Autodesk Inventor part; units mm, degrees
(part 3 of 3)
  line L372 (-9.4727, -16.9965) -> (-8.9155, -16.4393) projected
  line L373 (-10.552, -17.5763) -> (-10.5765, -17.5519) projected
  line L374 (-10.5765, -17.5519) -> (-10.9223, -17.8977) projected
  line L375 (-13.8024, -11.0005) -> (-15.4197, -12.6178) projected
  line L376 (-15.4197, -12.6178) -> (-15.1472, -12.8903) projected
  line L377 (-15.1472, -12.8903) -> (-13.5299, -11.273) projected
  line L378 (-13.5299, -11.273) -> (-13.8024, -11.0005) projected
  line L379 (-16.2092, -10.5708) -> (-15.3551, -11.4249) projected
  line L380 (-15.5559, -9.4461) -> (-15.8529, -9.743) projected
  line L381 (-15.8529, -9.743) -> (-15.8371, -9.7587) projected
  line L382 (-15.1472, -11.2171) -> (-16.2668, -10.0975) projected
  line L383 (-16.2668, -10.0975) -> (-16.4152, -10.246) projected
  line L384 (-16.0397, -8.7632) -> (-18.2911, -11.0145) projected
  line L385 (-18.2911, -11.0145) -> (-18.0186, -11.2869) projected
  line L386 (-18.0186, -11.2869) -> (-15.7673, -9.0356) projected
  line L387 (-15.7673, -9.0356) -> (-16.0397, -8.7632) projected
  circle A0 centre (-12.4372, -30.0261) radius 2.75 projected
  circle A1 centre (12.4372, -30.0261) radius 2.75 projected
  circle A2 centre (30.0261, -12.4372) radius 2.75 projected
  circle A3 centre (30.0261, 12.4372) radius 2.75 projected
  circle A4 centre (12.4372, 30.0261) radius 2.75 projected
  circle A5 centre (-22.981, 22.981) radius 2.75 projected
  circle A6 centre (-32.5, 0) radius 2.75 projected
  circle A7 centre (0, 32.5) radius 2.75 projected
  circle A8 centre (-30.0261, -12.4372) radius 2.75 projected
  circle A9 centre (-30.0261, 12.4372) radius 2.75 projected
  circle A10 centre (-12.4372, 30.0261) radius 2.75 projected
  circle A11 centre (22.981, 22.981) radius 2.75 projected
  circle A12 centre (32.5, 0) radius 2.75 projected
  circle A13 centre (22.981, -22.981) radius 2.75 projected
  circle A14 centre (0, -32.5) radius 2.75 projected
  circle A15 centre (-22.981, -22.981) radius 2.75 projected
  circle A16 centre (8, 0) radius 2.1 projected
  circle A17 centre (-8, 0) radius 2.1 projected
  circle A18 centre (0, -8) radius 2.1 projected
  circle A19 centre (0, 8) radius 2.1 projected
  circle A20 centre (0, 0) radius 40 projected
  point P0 (-18.4989, -9.1823)
  point P1 (-18.6788, -8.7509)
  point P2 (-18.0483, -9.3779)
  point P3 (-17.1051, -7.6244)
  point P4 (-17.4562, -7.3642)
  point P5 (-17.7426, -7.6052)
  point P6 (-17.3392, -7.8654)
  point P7 (-19.0264, -8.7422)
  point P8 (-18.7382, -9.3902)
  point P9 (-17.1278, -9.2749)
  point P10 (-14.8206, -13.2169)
  point P11 (-14.4905, -12.9881)
  point P12 (-12.9239, -14.6875)
  point P13 (-12.7055, -13.7251)
  point P14 (-11.6454, -13.5557)
  point P15 (-13.0077, -13.4649)
  point P16 (-13.247, -14.8814)
  point P17 (-11.4533, -13.2588)
  point P18 (-10.4577, -15.9066)
  point P19 (-9.9407, -15.2743)
  point P20 (-9.9145, -15.8629)
  point P21 (-11.7938, -16.0795)
  point P22 (-11.4271, -16.6873)
  point P23 (-11.1843, -16.448)
  point P24 (-11.4131, -16.111)
  point P25 (-10.3826, -16.3031)
  point P26 (-9.6141, -16.1249)
  point P27 (-9.3871, -15.6114)
  point P28 (-9.5914, -15.1206)
  point P29 (-9.9984, -14.8709)
  point P30 (-17.5317, -14.3054)
  point P31 (-17.8374, -14.4749)
  point P32 (-17.7099, -14.805)
  point P33 (6.0632, -18.84)
  point P34 (6.2413, -19.9019)
  point P35 (5.1811, -19.722)
  point P36 (5.0013, -18.6619)
  point P37 (4.9, -20.0032)
  point P38 (6.4754, -20.136)
  point P39 (6.3444, -18.5588)
  point P40 (4.7672, -18.4278)
  point P41 (7.8551, -18.2567)
  point P42 (6.7199, -16.9922)
  point P43 (7.691, -17.1983)
  point P44 (8.1503, -18.461)
  point P45 (8.4018, -17.7589)
  point P46 (7.9669, -16.9118)
  point P47 (7.1757, -16.4525)
  point P48 (6.5243, -16.6708)
  point P49 (6.3182, -16.9922)
  point P50 (12.2355, -14.3758)
  point P51 (12.0486, -14.0457)
  point P52 (11.6749, -14.1784)
  point P53 (13.5874, -11.3158)
  point P54 (13.7655, -12.3777)
  point P55 (12.7054, -12.1978)
  point P56 (12.5255, -11.1377)
  point P57 (12.4242, -12.479)
  point P58 (13.9996, -12.6118)
  point P59 (13.8686, -11.0346)
  point P60 (12.2914, -10.9036)
  point P61 (15.3235, -10.8408)
  point P62 (14.8921, -11.0207)
  point P63 (15.5191, -10.3901)
  point P64 (13.7655, -9.447)
  point P65 (13.5053, -9.7981)
  point P66 (13.7463, -10.0845)
  point P67 (14.0065, -9.681)
  point P68 (14.8833, -11.3682)
  point P69 (15.5313, -11.08)
  point P70 (15.416, -9.4697)
  point P71 (12.2779, -18.0318)
  point P72 (12.0543, -18.3392)
  point P73 (12.5207, -18.2641)
  point P74 (13.593, -18.4003)
  point P75 (13.7363, -19.4797)
  point P76 (13.3835, -19.6893)
  point P77 (13.9686, -19.7225)
  point P78 (14.2934, -18.9575)
  point P79 (13.8742, -18.1191)
  point P80 (13.0306, -17.6947)
  point P81 (16.9237, -13.3824)
  point P82 (16.557, -14.1405)
  point P83 (16.8189, -14.7937)
  point P84 (17.79, -14.9089)
  point P85 (18.3454, -14.5806)
  point P86 (18.962, -14.6347)
  point P87 (18.8554, -15.4189)
  point P88 (19.1227, -15.6477)
  point P89 (19.231, -14.3064)
  point P90 (18.7017, -14.0566)
  point P91 (18.1551, -14.2225)
  point P92 (17.6678, -14.5142)
  point P93 (17.0722, -14.4496)
  point P94 (17.1927, -13.6095)
  point P95 (19.6425, 8.1843)
  point P96 (19.8224, 7.7529)
  point P97 (19.1919, 8.3799)
  point P98 (18.2487, 6.6263)
  point P99 (18.5998, 6.3661)
  point P100 (18.8862, 6.6071)
  point P101 (18.4828, 6.8674)
  point P102 (20.17, 7.7441)
  point P103 (19.8818, 8.3921)
  point P104 (18.2714, 8.2768)
  point P105 (14.4727, 10.9019)
  point P106 (14.3399, 11.2757)
  point P107 (13.9277, 11.2198)
  point P108 (14.1426, 10.7151)
  point P109 (11.4913, 16.5067)
  point P110 (11.2904, 16.9835)
  point P111 (10.5167, 17.1983)
  point P112 (10.3735, 17.9004)
  point P113 (10.0451, 17.7118)
  point P114 (10.1586, 17.3712)
  point P115 (10.3839, 16.9712)
  point P116 (10.9621, 16.7948)
  point P117 (11.0756, 16.4543)
  point P118 (19.56, 15.8111)
  point P119 (19.2299, 15.6242)
  point P120 (19.3626, 15.2504)
  point P121 (16.7742, 16.8328)
  point P122 (16.2572, 16.2006)
  point P123 (16.231, 16.7892)
  point P124 (18.1103, 17.0057)
  point P125 (17.7435, 17.6135)
  point P126 (17.5008, 17.3743)
  point P127 (17.7296, 17.0372)
  point P128 (16.6991, 17.2293)
  point P129 (15.9306, 17.0512)
  point P130 (15.7035, 16.5377)
  point P131 (15.9079, 16.0469)
  point P132 (16.3148, 15.7971)
  point P133 (-9.5805, 14.9827)
  point P134 (-9.7587, 16.0446)
  point P135 (-8.6985, 15.8647)
  point P136 (-8.5186, 14.8046)
  point P137 (-8.4173, 16.1459)
  point P138 (-9.9927, 16.2787)
  point P139 (-9.8617, 14.7015)
  point P140 (-8.2846, 14.5705)
  point P141 (-11.2799, 14.4745)
  point P142 (-10.3228, 14.2649)
  point P143 (-10.1604, 13.2117)
  point P144 (-10.0731, 14.5775)
  point P145 (-11.4721, 14.7993)
  point P146 (-9.8704, 13.0126)
  point P147 (-12.9182, 12.8362)
  point P148 (-11.9611, 12.6266)
  point P149 (-11.7987, 11.5734)
  point P150 (-11.7113, 12.9392)
  point P151 (-13.1103, 13.161)
  point P152 (-11.5087, 11.3743)
  point P153 (-11.2804, 22.0882)
  point P154 (-11.0935, 21.7581)
  point P155 (-10.7197, 21.8908)
  point P156 (-12.7597, 20.1617)
  point P157 (-12.3283, 20.3416)
  point P158 (-12.9553, 19.7111)
  point P159 (-11.2018, 18.768)
  point P160 (-10.9415, 19.119)
  point P161 (-11.1826, 19.4054)
  point P162 (-11.4428, 19.002)
  point P163 (-12.3196, 20.6892)
  point P164 (-12.9675, 20.401)
  point P165 (-12.8523, 18.7907)
  point P166 (-18.5845, 13.02)
  point P167 (-17.9522, 12.503)
  point P168 (-18.5408, 12.4768)
  point P169 (-18.7574, 14.3561)
  point P170 (-19.3652, 13.9893)
  point P171 (-19.1259, 13.7466)
  point P172 (-18.7888, 13.9754)
  point P173 (-18.981, 12.9449)
  point P174 (-18.8028, 12.1764)
  point P175 (-18.2893, 11.9494)
  point P176 (-17.7985, 12.1537)
  point P177 (-17.5488, 12.5607)
  point P178 (-20.6542, 12.2148)
  point P179 (-19.5189, 10.9503)
  point P180 (-20.49, 11.1564)
  point P181 (-20.9493, 12.4192)
  point P182 (-21.2009, 11.7171)
  point P183 (-20.766, 10.87)
  point P184 (-19.9748, 10.4106)
  point P185 (-19.3233, 10.629)
  point P186 (-19.1172, 10.9503)
  point P187 (-21.779, 9.8255)
  point P188 (-21.1467, 9.3086)
  point P189 (-21.7353, 9.2824)
  point P190 (-21.9519, 11.1617)
  point P191 (-22.5597, 10.7949)
  point P192 (-22.3204, 10.5521)
  point P193 (-21.9833, 10.7809)
  point P194 (-22.1754, 9.7504)
  point P195 (-21.9973, 8.9819)
  point P196 (-21.4838, 8.7549)
  point P197 (-20.993, 8.9592)
  point P198 (-20.7433, 9.3662)
  point P199 (-24.0425, 9.7103)
  constraints: 429 other
